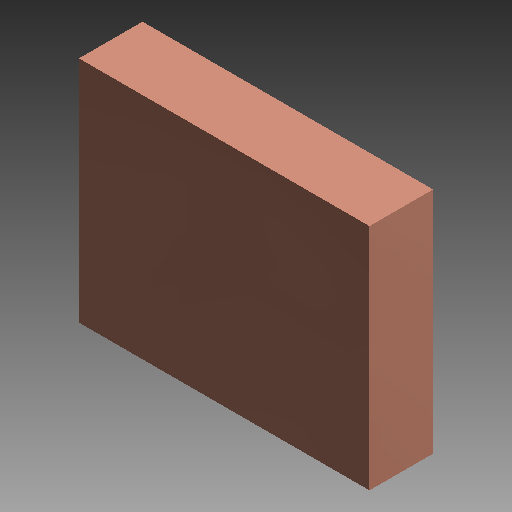
# Autodesk Inventor part: 7M-16.000MEEQ-T
Saved by Autodesk Inventor 2018.2 (Build 222227000, 227)
## iProperties
Part Number: 7M-16.000MEEQ-T
Material: Generic
Document SubType Name: Modeling
Designer: autocad
Appearance: CRYS320250, 7M-16.000MEEQ-T
Author: autocad
Autodesk Inventor part; units mm, degrees
ref_plane "YZ Plane" through (0, 0, 0) normal (1, 0, 0) x (0, 1, 0)
ref_plane "XZ Plane" through (0, 0, 0) normal (0, 1, 0) x (-1, 0, 0)
ref_plane "XY Plane" through (0, 0, 0) normal (0, 0, 1) x (1, 0, 0)
sketch "CRYS320250, 7M-16.000MEEQ-T_211" plane through (0, 0, 0) normal (0, 0, 1) x (1, 0, 0)
  line L0 (-1.5995, -1.2495) -> (-1.5995, 1.2695)
  line L1 (-1.5995, 1.2695) -> (1.5997, 1.2695)
  line L2 (1.5997, 1.2695) -> (1.5997, -1.2495)
  line L3 (1.5997, -1.2495) -> (-1.5995, -1.2495)
  constraints: 8 end point
extrude "Extrusion1" add sketch "CRYS320250, 7M-16.000MEEQ-T_211" along normal blind 0.7
body "Solid1"
